Autodesk Fusion 360 part; units mm, degrees
(part 7 of 9)
equation "d395 = ( BaseX + TowerWidth + ModuleGap ) + ( ( ( LeftRun - TowerWidth - ModuleGap ) / 2 ) - DrainWidth / 2 )"
equation "d397 = -( -( ( FootHeight ) + FloorMin + DrainExtension * tan(DrainSlope) + ( ( Depth ) - ( ( Depth ) - Wall ) ) * tan(DrainSlope) ) )"
equation "d398 = ( ( BaseY ) + ( ( Depth ) - Wall ) )"
equation "d399 = -( -( ( FootHeight ) + FloorMin + DrainExtension * tan(DrainSlope) + ( ( Depth ) - ( ( Depth ) + DrainExtension ) ) * tan(DrainSlope) ) )"
equation "d400 = ( ( BaseY ) + ( ( Depth ) + DrainExtension ) )"
equation "d401 = -( -( ( FootHeight ) + PanHeight + 1 mm ) )"
equation "d402 = DrainWidth"
equation "d404 = FootHeight"
equation "d406 = ( BaseX + TowerWidth + ModuleGap ) + ( Wall )"
equation "d407 = ( BaseY ) + ( Wall )"
equation "d410 = PanHeight - DeckThick"
equation "d412 = FootHeight"
equation "d414 = ( BaseX + TowerWidth + ModuleGap ) + ( Wall )"
equation "d415 = ( BaseY ) + ( ( Depth ) - Wall - 12 mm )"
equation "d418 = PanHeight - DeckThick"
equation "d420 = FootHeight"
equation "d422 = ( BaseX + TowerWidth + ModuleGap ) + ( ( LeftRun - TowerWidth - ModuleGap ) - Wall - 12 mm )"
equation "d423 = ( BaseY ) + ( Wall )"
equation "d426 = PanHeight - DeckThick"
equation "d428 = FootHeight"
equation "d430 = ( BaseX + TowerWidth + ModuleGap ) + ( ( LeftRun - TowerWidth - ModuleGap ) - Wall - 12 mm )"
equation "d431 = ( BaseY ) + ( ( Depth ) - Wall - 12 mm )"
equation "d434 = PanHeight - DeckThick"
equation "d436 = ( BaseX + TowerWidth + ModuleGap ) + ( ( ( LeftRun - TowerWidth - ModuleGap ) / 2 ) - DrainWidth / 2 - Wall )"
equation "d438 = -( -( ( FootHeight ) - ( 0.2 mm ) ) )"
equation "d439 = ( ( BaseY ) + ( ( Depth ) + DrainExtension - 2 mm ) )"
equation "d440 = ( ( BaseY ) + ( ( ( Depth ) + DrainExtension - 2 mm ) + ( 1 mm ) ) )"
equation "d441 = -( -( ( FootHeight ) + ( 0.6 mm ) ) )"
equation "d442 = DrainWidth + 2 * Wall"
equation "d444 = FootHeight"
equation "d446 = ( BaseX + TowerWidth + ModuleGap ) + ( ( 11 mm ) - PegSize / 2 - FitClearance )"
equation "d447 = ( BaseY ) + ( ( 11 mm ) - PegSize / 2 - FitClearance )"
equation "d448 = PegSize + 2 * FitClearance"
equation "d449 = PegSize + 2 * FitClearance"
equation "d450 = PegHeight + 0.3 mm"
equation "d452 = FootHeight"
equation "d454 = ( BaseX + TowerWidth + ModuleGap ) + ( ( 11 mm ) - PegSize / 2 - FitClearance )"
equation "d455 = ( BaseY ) + ( ( ( Depth ) - FrontFootInset ) - PegSize / 2 - FitClearance )"
equation "d456 = PegSize + 2 * FitClearance"
equation "d457 = PegSize + 2 * FitClearance"
equation "d458 = PegHeight + 0.3 mm"
equation "d460 = FootHeight"
equation "d462 = ( BaseX + TowerWidth + ModuleGap ) + ( ( ( LeftRun - TowerWidth - ModuleGap ) - 11 mm ) - PegSize / 2 - FitClearance )"
equation "d463 = ( BaseY ) + ( ( 11 mm ) - PegSize / 2 - FitClearance )"
equation "d464 = PegSize + 2 * FitClearance"
equation "d465 = PegSize + 2 * FitClearance"
equation "d466 = PegHeight + 0.3 mm"
equation "d468 = FootHeight"
equation "d470 = ( BaseX + TowerWidth + ModuleGap ) + ( ( ( LeftRun - TowerWidth - ModuleGap ) - 11 mm ) - PegSize / 2 - FitClearance )"
equation "d471 = ( BaseY ) + ( ( ( Depth ) - FrontFootInset ) - PegSize / 2 - FitClearance )"
equation "d472 = PegSize + 2 * FitClearance"
equation "d473 = PegSize + 2 * FitClearance"
equation "d474 = PegHeight + 0.3 mm"
equation "d476 = ( FootHeight ) + PanHeight - DeckThick"
equation "d478 = ( BaseX + TowerWidth + ModuleGap ) + ( Wall + DeckClearance )"
equation "d479 = ( BaseY ) + ( Wall + DeckClearance )"
equation "d480 = ( LeftRun - TowerWidth - ModuleGap ) - 2 * ( Wall + DeckClearance )"
equation "d481 = ( Depth ) - 2 * ( Wall + DeckClearance )"
equation "d482 = DeckThick"
equation "d484 = ( FootHeight ) + PanHeight - DeckThick"
equation "d486 = ( BaseX + TowerWidth + ModuleGap ) + ( ( ( ( LeftRun - TowerWidth - ModuleGap ) - ( 16 * SlotPitch + SlotWidth ) ) / 2 ) + ( 0 * SlotPitch ) )"
equation "d487 = ( BaseY ) + ( Wall + DeckClearance + RimBorder )"
equation "d488 = SlotWidth"
equation "d489 = ( Depth ) - 2 * ( Wall + DeckClearance + RimBorder )"
equation "d490 = DeckThick"
equation "d492 = ( FootHeight ) + PanHeight - DeckThick"
equation "d494 = ( BaseX + TowerWidth + ModuleGap ) + ( ( ( ( LeftRun - TowerWidth - ModuleGap ) - ( 16 * SlotPitch + SlotWidth ) ) / 2 ) + ( 1 * SlotPitch ) )"
equation "d495 = ( BaseY ) + ( Wall + DeckClearance + RimBorder )"
equation "d496 = SlotWidth"
equation "d497 = ( Depth ) - 2 * ( Wall + DeckClearance + RimBorder )"
equation "d498 = DeckThick"
equation "d500 = ( FootHeight ) + PanHeight - DeckThick"
equation "d502 = ( BaseX + TowerWidth + ModuleGap ) + ( ( ( ( LeftRun - TowerWidth - ModuleGap ) - ( 16 * SlotPitch + SlotWidth ) ) / 2 ) + ( 2 * SlotPitch ) )"
equation "d503 = ( BaseY ) + ( Wall + DeckClearance + RimBorder )"
equation "d504 = SlotWidth"
equation "d505 = ( Depth ) - 2 * ( Wall + DeckClearance + RimBorder )"
equation "d506 = DeckThick"
equation "d508 = ( FootHeight ) + PanHeight - DeckThick"
equation "d510 = ( BaseX + TowerWidth + ModuleGap ) + ( ( ( ( LeftRun - TowerWidth - ModuleGap ) - ( 16 * SlotPitch + SlotWidth ) ) / 2 ) + ( 3 * SlotPitch ) )"
equation "d511 = ( BaseY ) + ( Wall + DeckClearance + RimBorder )"
equation "d512 = SlotWidth"
equation "d513 = ( Depth ) - 2 * ( Wall + DeckClearance + RimBorder )"
equation "d514 = DeckThick"
equation "d516 = ( FootHeight ) + PanHeight - DeckThick"
equation "d518 = ( BaseX + TowerWidth + ModuleGap ) + ( ( ( ( LeftRun - TowerWidth - ModuleGap ) - ( 16 * SlotPitch + SlotWidth ) ) / 2 ) + ( 4 * SlotPitch ) )"
equation "d519 = ( BaseY ) + ( Wall + DeckClearance + RimBorder )"
equation "d520 = SlotWidth"
equation "d521 = ( Depth ) - 2 * ( Wall + DeckClearance + RimBorder )"
equation "d522 = DeckThick"
equation "d524 = ( FootHeight ) + PanHeight - DeckThick"
equation "d526 = ( BaseX + TowerWidth + ModuleGap ) + ( ( ( ( LeftRun - TowerWidth - ModuleGap ) - ( 16 * SlotPitch + SlotWidth ) ) / 2 ) + ( 5 * SlotPitch ) )"
equation "d527 = ( BaseY ) + ( Wall + DeckClearance + RimBorder )"
equation "d528 = SlotWidth"
equation "d529 = ( Depth ) - 2 * ( Wall + DeckClearance + RimBorder )"
equation "d530 = DeckThick"
equation "d532 = ( FootHeight ) + PanHeight - DeckThick"
equation "d534 = ( BaseX + TowerWidth + ModuleGap ) + ( ( ( ( LeftRun - TowerWidth - ModuleGap ) - ( 16 * SlotPitch + SlotWidth ) ) / 2 ) + ( 6 * SlotPitch ) )"
equation "d535 = ( BaseY ) + ( Wall + DeckClearance + RimBorder )"
equation "d536 = SlotWidth"
equation "d537 = ( Depth ) - 2 * ( Wall + DeckClearance + RimBorder )"
equation "d538 = DeckThick"
equation "d540 = ( FootHeight ) + PanHeight - DeckThick"
equation "d542 = ( BaseX + TowerWidth + ModuleGap ) + ( ( ( ( LeftRun - TowerWidth - ModuleGap ) - ( 16 * SlotPitch + SlotWidth ) ) / 2 ) + ( 7 * SlotPitch ) )"
equation "d543 = ( BaseY ) + ( Wall + DeckClearance + RimBorder )"
equation "d544 = SlotWidth"
equation "d545 = ( Depth ) - 2 * ( Wall + DeckClearance + RimBorder )"
equation "d546 = DeckThick"
equation "d548 = ( FootHeight ) + PanHeight - DeckThick"
equation "d550 = ( BaseX + TowerWidth + ModuleGap ) + ( ( ( ( LeftRun - TowerWidth - ModuleGap ) - ( 16 * SlotPitch + SlotWidth ) ) / 2 ) + ( 8 * SlotPitch ) )"
equation "d551 = ( BaseY ) + ( Wall + DeckClearance + RimBorder )"
equation "d552 = SlotWidth"
equation "d553 = ( Depth ) - 2 * ( Wall + DeckClearance + RimBorder )"
equation "d554 = DeckThick"
equation "d556 = ( FootHeight ) + PanHeight - DeckThick"
equation "d558 = ( BaseX + TowerWidth + ModuleGap ) + ( ( ( ( LeftRun - TowerWidth - ModuleGap ) - ( 16 * SlotPitch + SlotWidth ) ) / 2 ) + ( 9 * SlotPitch ) )"
equation "d559 = ( BaseY ) + ( Wall + DeckClearance + RimBorder )"
equation "d560 = SlotWidth"
equation "d561 = ( Depth ) - 2 * ( Wall + DeckClearance + RimBorder )"
equation "d562 = DeckThick"
equation "d564 = ( FootHeight ) + PanHeight - DeckThick"
equation "d566 = ( BaseX + TowerWidth + ModuleGap ) + ( ( ( ( LeftRun - TowerWidth - ModuleGap ) - ( 16 * SlotPitch + SlotWidth ) ) / 2 ) + ( 10 * SlotPitch ) )"
equation "d567 = ( BaseY ) + ( Wall + DeckClearance + RimBorder )"
equation "d568 = SlotWidth"
equation "d569 = ( Depth ) - 2 * ( Wall + DeckClearance + RimBorder )"
equation "d570 = DeckThick"
equation "d572 = ( FootHeight ) + PanHeight - DeckThick"
equation "d574 = ( BaseX + TowerWidth + ModuleGap ) + ( ( ( ( LeftRun - TowerWidth - ModuleGap ) - ( 16 * SlotPitch + SlotWidth ) ) / 2 ) + ( 11 * SlotPitch ) )"
equation "d575 = ( BaseY ) + ( Wall + DeckClearance + RimBorder )"
equation "d576 = SlotWidth"
equation "d577 = ( Depth ) - 2 * ( Wall + DeckClearance + RimBorder )"
equation "d578 = DeckThick"
equation "d580 = ( FootHeight ) + PanHeight - DeckThick"
equation "d582 = ( BaseX + TowerWidth + ModuleGap ) + ( ( ( ( LeftRun - TowerWidth - ModuleGap ) - ( 16 * SlotPitch + SlotWidth ) ) / 2 ) + ( 12 * SlotPitch ) )"
equation "d583 = ( BaseY ) + ( Wall + DeckClearance + RimBorder )"
equation "d584 = SlotWidth"
equation "d585 = ( Depth ) - 2 * ( Wall + DeckClearance + RimBorder )"
equation "d586 = DeckThick"
equation "d588 = ( FootHeight ) + PanHeight - DeckThick"
equation "d590 = ( BaseX + TowerWidth + ModuleGap ) + ( ( ( ( LeftRun - TowerWidth - ModuleGap ) - ( 16 * SlotPitch + SlotWidth ) ) / 2 ) + ( 13 * SlotPitch ) )"
equation "d591 = ( BaseY ) + ( Wall + DeckClearance + RimBorder )"
equation "d592 = SlotWidth"
equation "d593 = ( Depth ) - 2 * ( Wall + DeckClearance + RimBorder )"
equation "d594 = DeckThick"
equation "d596 = ( FootHeight ) + PanHeight - DeckThick"
equation "d598 = ( BaseX + TowerWidth + ModuleGap ) + ( ( ( ( LeftRun - TowerWidth - ModuleGap ) - ( 16 * SlotPitch + SlotWidth ) ) / 2 ) + ( 14 * SlotPitch ) )"
equation "d599 = ( BaseY ) + ( Wall + DeckClearance + RimBorder )"
equation "d600 = SlotWidth"
equation "d601 = ( Depth ) - 2 * ( Wall + DeckClearance + RimBorder )"
equation "d602 = DeckThick"
equation "d604 = ( FootHeight ) + PanHeight - DeckThick"
equation "d606 = ( BaseX + TowerWidth + ModuleGap ) + ( ( ( ( LeftRun - TowerWidth - ModuleGap ) - ( 16 * SlotPitch + SlotWidth ) ) / 2 ) + ( 15 * SlotPitch ) )"
equation "d607 = ( BaseY ) + ( Wall + DeckClearance + RimBorder )"
equation "d608 = SlotWidth"
equation "d609 = ( Depth ) - 2 * ( Wall + DeckClearance + RimBorder )"
equation "d610 = DeckThick"
equation "d612 = ( FootHeight ) + PanHeight - DeckThick"
equation "d614 = ( BaseX + TowerWidth + ModuleGap ) + ( ( ( ( LeftRun - TowerWidth - ModuleGap ) - ( 16 * SlotPitch + SlotWidth ) ) / 2 ) + ( 16 * SlotPitch ) )"
equation "d615 = ( BaseY ) + ( Wall + DeckClearance + RimBorder )"
equation "d616 = SlotWidth"
equation "d617 = ( Depth ) - 2 * ( Wall + DeckClearance + RimBorder )"
equation "d618 = DeckThick"
equation "d620 = ( FootHeight ) + PanHeight - DeckThick"
equation "d622 = ( BaseX + TowerWidth + ModuleGap ) + ( ( LeftRun - TowerWidth - ModuleGap ) / 2 - 8 mm )"
equation "d623 = ( BaseY ) + ( ( Depth ) - Wall - DeckClearance - 4 mm )"
equation "d626 = DeckThick"
equation "d630 = ( BaseX + TowerWidth + ModuleGap ) + ( ( 11 mm ) - FootSize / 2 )"
equation "d631 = ( BaseY ) + ( ( 11 mm ) - FootSize / 2 )"
equation "d632 = FootSize"
equation "d633 = FootSize"
equation "d634 = FootHeight"
equation "d636 = FootHeight"
equation "d638 = ( BaseX + TowerWidth + ModuleGap ) + ( ( 11 mm ) - PegSize / 2 )"
equation "d639 = ( BaseY ) + ( ( 11 mm ) - PegSize / 2 )"
equation "d640 = PegSize"
equation "d641 = PegSize"
equation "d642 = PegHeight"
equation "d646 = ( BaseX + TowerWidth + ModuleGap ) + ( ( 11 mm ) - FootSize / 2 )"
equation "d647 = ( BaseY ) + ( ( ( Depth ) - FrontFootInset ) - FootSize / 2 )"
equation "d648 = FootSize"
equation "d649 = FootSize"
equation "d650 = FootHeight"
equation "d652 = FootHeight"
equation "d654 = ( BaseX + TowerWidth + ModuleGap ) + ( ( 11 mm ) - PegSize / 2 )"
equation "d655 = ( BaseY ) + ( ( ( Depth ) - FrontFootInset ) - PegSize / 2 )"
equation "d656 = PegSize"
equation "d657 = PegSize"
equation "d658 = PegHeight"
equation "d662 = ( BaseX + TowerWidth + ModuleGap ) + ( ( ( LeftRun - TowerWidth - ModuleGap ) - 11 mm ) - FootSize / 2 )"
equation "d663 = ( BaseY ) + ( ( 11 mm ) - FootSize / 2 )"
equation "d664 = FootSize"
equation "d665 = FootSize"
equation "d666 = FootHeight"
equation "d668 = FootHeight"
equation "d670 = ( BaseX + TowerWidth + ModuleGap ) + ( ( ( LeftRun - TowerWidth - ModuleGap ) - 11 mm ) - PegSize / 2 )"
equation "d671 = ( BaseY ) + ( ( 11 mm ) - PegSize / 2 )"
equation "d672 = PegSize"
equation "d673 = PegSize"
equation "d674 = PegHeight"
equation "d678 = ( BaseX + TowerWidth + ModuleGap ) + ( ( ( LeftRun - TowerWidth - ModuleGap ) - 11 mm ) - FootSize / 2 )"
equation "d679 = ( BaseY ) + ( ( ( Depth ) - FrontFootInset ) - FootSize / 2 )"
equation "d680 = FootSize"
equation "d681 = FootSize"
equation "d682 = FootHeight"
equation "d684 = FootHeight"
equation "d686 = ( BaseX + TowerWidth + ModuleGap ) + ( ( ( LeftRun - TowerWidth - ModuleGap ) - 11 mm ) - PegSize / 2 )"
equation "d687 = ( BaseY ) + ( ( ( Depth ) - FrontFootInset ) - PegSize / 2 )"
equation "d688 = PegSize"
equation "d689 = PegSize"
equation "d690 = PegHeight"
equation "d692 = FootHeight"
equation "d694 = ( BaseX + LeftRun + FaucetGap ) + ( 0 mm )"
equation "d695 = ( BaseY ) + ( 0 mm )"
equation "d696 = ( RightRun - ModuleGap ) / 2"
equation "d697 = Depth"
equation "d698 = PanHeight"
equation "d702 = ( BaseX + LeftRun + FaucetGap ) + ( Wall )"
equation "d704 = -( -( ( FootHeight ) + FloorMin + DrainExtension * tan(DrainSlope) + ( ( Depth ) - ( Wall ) ) * tan(DrainSlope) ) )"
equation "d705 = ( ( BaseY ) + ( Wall ) )"
equation "d706 = -( -( ( FootHeight ) + FloorMin + DrainExtension * tan(DrainSlope) + ( ( Depth ) - ( ( Depth ) - Wall ) ) * tan(DrainSlope) ) )"
equation "d707 = ( ( BaseY ) + ( ( Depth ) - Wall ) )"
equation "d708 = -( -( ( FootHeight ) + PanHeight + 1 mm ) )"
equation "d709 = ( ( RightRun - ModuleGap ) / 2 ) - 2 * Wall"
equation "d711 = ( BaseX + LeftRun + FaucetGap ) + ( ( ( RightRun - ModuleGap ) / 4 ) - DrainWidth / 2 - Wall )"
equation "d713 = -( -( FootHeight ) )"
equation "d714 = ( ( BaseY ) + ( ( Depth ) - Wall ) )"
equation "d715 = ( ( BaseY ) + ( ( Depth ) + DrainExtension ) )"
equation "d716 = -( -( ( FootHeight ) + FloorMin + DrainExtension * tan(DrainSlope) + ( ( Depth ) - ( ( Depth ) + DrainExtension ) ) * tan(DrainSlope) ) )"
equation "d717 = -( -( ( FootHeight ) + FloorMin + DrainExtension * tan(DrainSlope) + ( ( Depth ) - ( ( Depth ) - Wall ) ) * tan(DrainSlope) ) )"
equation "d718 = DrainWidth + 2 * Wall"
equation "d720 = ( BaseX + LeftRun + FaucetGap ) + ( ( ( RightRun - ModuleGap ) / 4 ) - DrainWidth / 2 - Wall )"
equation "d722 = -( -( FootHeight ) )"
equation "d723 = ( ( BaseY ) + ( ( Depth ) - Wall ) )"
equation "d724 = ( ( BaseY ) + ( ( Depth ) + DrainExtension ) )"
equation "d725 = -( -( ( ( FootHeight ) + FloorMin + DrainExtension * tan(DrainSlope) + ( ( Depth ) - ( ( Depth ) + DrainExtension ) ) * tan(DrainSlope) ) + ( 6 mm ) ) )"
equation "d726 = -( -( ( ( FootHeight ) + FloorMin + DrainExtension * tan(DrainSlope) + ( ( Depth ) - ( ( Depth ) - Wall ) ) * tan(DrainSlope) ) + ( 6 mm ) ) )"
equation "d727 = Wall"
equation "d729 = ( BaseX + LeftRun + FaucetGap ) + ( ( ( RightRun - ModuleGap ) / 4 ) + DrainWidth / 2 )"
equation "d731 = -( -( FootHeight ) )"
equation "d732 = ( ( BaseY ) + ( ( Depth ) - Wall ) )"
equation "d733 = ( ( BaseY ) + ( ( Depth ) + DrainExtension ) )"
equation "d734 = -( -( ( ( FootHeight ) + FloorMin + DrainExtension * tan(DrainSlope) + ( ( Depth ) - ( ( Depth ) + DrainExtension ) ) * tan(DrainSlope) ) + ( 6 mm ) ) )"
equation "d735 = -( -( ( ( FootHeight ) + FloorMin + DrainExtension * tan(DrainSlope) + ( ( Depth ) - ( ( Depth ) - Wall ) ) * tan(DrainSlope) ) + ( 6 mm ) ) )"
equation "d736 = Wall"
equation "d738 = ( BaseX + LeftRun + FaucetGap ) + ( ( ( RightRun - ModuleGap ) / 4 ) - DrainWidth / 2 )"
equation "d740 = -( -( ( FootHeight ) + FloorMin + DrainExtension * tan(DrainSlope) + ( ( Depth ) - ( ( Depth ) - Wall ) ) * tan(DrainSlope) ) )"
equation "d741 = ( ( BaseY ) + ( ( Depth ) - Wall ) )"
equation "d742 = -( -( ( FootHeight ) + FloorMin + DrainExtension * tan(DrainSlope) + ( ( Depth ) - ( ( Depth ) + DrainExtension ) ) * tan(DrainSlope) ) )"
equation "d743 = ( ( BaseY ) + ( ( Depth ) + DrainExtension ) )"
equation "d744 = -( -( ( FootHeight ) + PanHeight + 1 mm ) )"
equation "d745 = DrainWidth"
equation "d747 = FootHeight"
equation "d749 = ( BaseX + LeftRun + FaucetGap ) + ( Wall )"
equation "d750 = ( BaseY ) + ( Wall )"
equation "d753 = PanHeight - DeckThick"
equation "d755 = FootHeight"
equation "d757 = ( BaseX + LeftRun + FaucetGap ) + ( Wall )"
equation "d758 = ( BaseY ) + ( ( Depth ) - Wall - 12 mm )"
equation "d761 = PanHeight - DeckThick"
equation "d763 = FootHeight"
equation "d765 = ( BaseX + LeftRun + FaucetGap ) + ( ( ( RightRun - ModuleGap ) / 2 ) - Wall - 12 mm )"
equation "d766 = ( BaseY ) + ( Wall )"
equation "d769 = PanHeight - DeckThick"
equation "d771 = FootHeight"
equation "d773 = ( BaseX + LeftRun + FaucetGap ) + ( ( ( RightRun - ModuleGap ) / 2 ) - Wall - 12 mm )"
equation "d774 = ( BaseY ) + ( ( Depth ) - Wall - 12 mm )"
equation "d777 = PanHeight - DeckThick"
equation "d779 = ( BaseX + LeftRun + FaucetGap ) + ( ( ( RightRun - ModuleGap ) / 4 ) - DrainWidth / 2 - Wall )"
equation "d781 = -( -( ( FootHeight ) - ( 0.2 mm ) ) )"
equation "d782 = ( ( BaseY ) + ( ( Depth ) + DrainExtension - 2 mm ) )"
equation "d783 = ( ( BaseY ) + ( ( ( Depth ) + DrainExtension - 2 mm ) + ( 1 mm ) ) )"
equation "d784 = -( -( ( FootHeight ) + ( 0.6 mm ) ) )"
equation "d785 = DrainWidth + 2 * Wall"
equation "d787 = FootHeight"
equation "d789 = ( BaseX + LeftRun + FaucetGap ) + ( ( 11 mm ) - PegSize / 2 - FitClearance )"
equation "d790 = ( BaseY ) + ( ( 11 mm ) - PegSize / 2 - FitClearance )"
equation "d791 = PegSize + 2 * FitClearance"
equation "d792 = PegSize + 2 * FitClearance"
equation "d793 = PegHeight + 0.3 mm"
equation "d795 = FootHeight"
equation "d797 = ( BaseX + LeftRun + FaucetGap ) + ( ( 11 mm ) - PegSize / 2 - FitClearance )"
equation "d798 = ( BaseY ) + ( ( ( Depth ) - FrontFootInset ) - PegSize / 2 - FitClearance )"
equation "d799 = PegSize + 2 * FitClearance"
equation "d800 = PegSize + 2 * FitClearance"
equation "d801 = PegHeight + 0.3 mm"
equation "d803 = FootHeight"
equation "d805 = ( BaseX + LeftRun + FaucetGap ) + ( ( ( ( RightRun - ModuleGap ) / 2 ) - 11 mm ) - PegSize / 2 - FitClearance )"
equation "d806 = ( BaseY ) + ( ( 11 mm ) - PegSize / 2 - FitClearance )"
equation "d807 = PegSize + 2 * FitClearance"
equation "d808 = PegSize + 2 * FitClearance"
equation "d809 = PegHeight + 0.3 mm"
equation "d811 = FootHeight"
equation "d813 = ( BaseX + LeftRun + FaucetGap ) + ( ( ( ( RightRun - ModuleGap ) / 2 ) - 11 mm ) - PegSize / 2 - FitClearance )"
equation "d814 = ( BaseY ) + ( ( ( Depth ) - FrontFootInset ) - PegSize / 2 - FitClearance )"
equation "d815 = PegSize + 2 * FitClearance"
equation "d816 = PegSize + 2 * FitClearance"
equation "d817 = PegHeight + 0.3 mm"
equation "d819 = ( FootHeight ) + PanHeight - DeckThick"
equation "d821 = ( BaseX + LeftRun + FaucetGap ) + ( Wall + DeckClearance )"
equation "d822 = ( BaseY ) + ( Wall + DeckClearance )"
equation "d823 = ( ( RightRun - ModuleGap ) / 2 ) - 2 * ( Wall + DeckClearance )"
equation "d824 = ( Depth ) - 2 * ( Wall + DeckClearance )"
equation "d825 = DeckThick"
equation "d827 = ( FootHeight ) + PanHeight - DeckThick"
equation "d829 = ( BaseX + LeftRun + FaucetGap ) + ( ( ( ( ( RightRun - ModuleGap ) / 2 ) - ( 10 * SlotPitch + SlotWidth ) ) / 2 ) + ( 0 * SlotPitch ) )"
equation "d830 = ( BaseY ) + ( Wall + DeckClearance + RimBorder )"
equation "d831 = SlotWidth"
equation "d832 = ( Depth ) - 2 * ( Wall + DeckClearance + RimBorder )"
equation "d833 = DeckThick"
equation "d835 = ( FootHeight ) + PanHeight - DeckThick"
equation "d837 = ( BaseX + LeftRun + FaucetGap ) + ( ( ( ( ( RightRun - ModuleGap ) / 2 ) - ( 10 * SlotPitch + SlotWidth ) ) / 2 ) + ( 1 * SlotPitch ) )"
equation "d838 = ( BaseY ) + ( Wall + DeckClearance + RimBorder )"
equation "d839 = SlotWidth"
equation "d840 = ( Depth ) - 2 * ( Wall + DeckClearance + RimBorder )"
equation "d841 = DeckThick"
equation "d843 = ( FootHeight ) + PanHeight - DeckThick"
equation "d845 = ( BaseX + LeftRun + FaucetGap ) + ( ( ( ( ( RightRun - ModuleGap ) / 2 ) - ( 10 * SlotPitch + SlotWidth ) ) / 2 ) + ( 2 * SlotPitch ) )"
equation "d846 = ( BaseY ) + ( Wall + DeckClearance + RimBorder )"
equation "d847 = SlotWidth"
equation "d848 = ( Depth ) - 2 * ( Wall + DeckClearance + RimBorder )"
equation "d849 = DeckThick"
equation "d851 = ( FootHeight ) + PanHeight - DeckThick"
equation "d853 = ( BaseX + LeftRun + FaucetGap ) + ( ( ( ( ( RightRun - ModuleGap ) / 2 ) - ( 10 * SlotPitch + SlotWidth ) ) / 2 ) + ( 3 * SlotPitch ) )"
equation "d854 = ( BaseY ) + ( Wall + DeckClearance + RimBorder )"
equation "d855 = SlotWidth"
equation "d856 = ( Depth ) - 2 * ( Wall + DeckClearance + RimBorder )"
equation "d857 = DeckThick"
equation "d859 = ( FootHeight ) + PanHeight - DeckThick"
equation "d861 = ( BaseX + LeftRun + FaucetGap ) + ( ( ( ( ( RightRun - ModuleGap ) / 2 ) - ( 10 * SlotPitch + SlotWidth ) ) / 2 ) + ( 4 * SlotPitch ) )"
equation "d862 = ( BaseY ) + ( Wall + DeckClearance + RimBorder )"
equation "d863 = SlotWidth"
equation "d864 = ( Depth ) - 2 * ( Wall + DeckClearance + RimBorder )"
equation "d865 = DeckThick"
equation "d867 = ( FootHeight ) + PanHeight - DeckThick"
equation "d869 = ( BaseX + LeftRun + FaucetGap ) + ( ( ( ( ( RightRun - ModuleGap ) / 2 ) - ( 10 * SlotPitch + SlotWidth ) ) / 2 ) + ( 5 * SlotPitch ) )"
equation "d870 = ( BaseY ) + ( Wall + DeckClearance + RimBorder )"
equation "d871 = SlotWidth"
equation "d872 = ( Depth ) - 2 * ( Wall + DeckClearance + RimBorder )"
equation "d873 = DeckThick"
equation "d875 = ( FootHeight ) + PanHeight - DeckThick"
equation "d877 = ( BaseX + LeftRun + FaucetGap ) + ( ( ( ( ( RightRun - ModuleGap ) / 2 ) - ( 10 * SlotPitch + SlotWidth ) ) / 2 ) + ( 6 * SlotPitch ) )"
equation "d878 = ( BaseY ) + ( Wall + DeckClearance + RimBorder )"
equation "d879 = SlotWidth"
equation "d880 = ( Depth ) - 2 * ( Wall + DeckClearance + RimBorder )"
equation "d881 = DeckThick"
equation "d883 = ( FootHeight ) + PanHeight - DeckThick"
equation "d885 = ( BaseX + LeftRun + FaucetGap ) + ( ( ( ( ( RightRun - ModuleGap ) / 2 ) - ( 10 * SlotPitch + SlotWidth ) ) / 2 ) + ( 7 * SlotPitch ) )"
equation "d886 = ( BaseY ) + ( Wall + DeckClearance + RimBorder )"
equation "d887 = SlotWidth"
equation "d888 = ( Depth ) - 2 * ( Wall + DeckClearance + RimBorder )"
equation "d889 = DeckThick"
equation "d891 = ( FootHeight ) + PanHeight - DeckThick"
equation "d893 = ( BaseX + LeftRun + FaucetGap ) + ( ( ( ( ( RightRun - ModuleGap ) / 2 ) - ( 10 * SlotPitch + SlotWidth ) ) / 2 ) + ( 8 * SlotPitch ) )"
equation "d894 = ( BaseY ) + ( Wall + DeckClearance + RimBorder )"
equation "d895 = SlotWidth"
equation "d896 = ( Depth ) - 2 * ( Wall + DeckClearance + RimBorder )"
equation "d897 = DeckThick"
equation "d899 = ( FootHeight ) + PanHeight - DeckThick"
equation "d901 = ( BaseX + LeftRun + FaucetGap ) + ( ( ( ( ( RightRun - ModuleGap ) / 2 ) - ( 10 * SlotPitch + SlotWidth ) ) / 2 ) + ( 9 * SlotPitch ) )"
equation "d902 = ( BaseY ) + ( Wall + DeckClearance + RimBorder )"
equation "d903 = SlotWidth"
equation "d904 = ( Depth ) - 2 * ( Wall + DeckClearance + RimBorder )"
equation "d905 = DeckThick"
equation "d907 = ( FootHeight ) + PanHeight - DeckThick"
equation "d909 = ( BaseX + LeftRun + FaucetGap ) + ( ( ( ( ( RightRun - ModuleGap ) / 2 ) - ( 10 * SlotPitch + SlotWidth ) ) / 2 ) + ( 10 * SlotPitch ) )"
equation "d910 = ( BaseY ) + ( Wall + DeckClearance + RimBorder )"
equation "d911 = SlotWidth"
equation "d912 = ( Depth ) - 2 * ( Wall + DeckClearance + RimBorder )"
equation "d913 = DeckThick"
equation "d915 = ( FootHeight ) + PanHeight - DeckThick"
equation "d917 = ( BaseX + LeftRun + FaucetGap ) + ( ( ( RightRun - ModuleGap ) / 2 ) / 2 - 8 mm )"
equation "d918 = ( BaseY ) + ( ( Depth ) - Wall - DeckClearance - 4 mm )"
equation "d921 = DeckThick"
equation "d925 = ( BaseX + LeftRun + FaucetGap ) + ( ( 11 mm ) - FootSize / 2 )"
equation "d926 = ( BaseY ) + ( ( 11 mm ) - FootSize / 2 )"
equation "d927 = FootSize"
equation "d928 = FootSize"
equation "d929 = FootHeight"
equation "d931 = FootHeight"
equation "d933 = ( BaseX + LeftRun + FaucetGap ) + ( ( 11 mm ) - PegSize / 2 )"
equation "d934 = ( BaseY ) + ( ( 11 mm ) - PegSize / 2 )"
equation "d935 = PegSize"
equation "d936 = PegSize"
equation "d937 = PegHeight"
equation "d941 = ( BaseX + LeftRun + FaucetGap ) + ( ( 11 mm ) - FootSize / 2 )"
equation "d942 = ( BaseY ) + ( ( ( Depth ) - FrontFootInset ) - FootSize / 2 )"
equation "d943 = FootSize"
equation "d944 = FootSize"
equation "d945 = FootHeight"
equation "d947 = FootHeight"
equation "d949 = ( BaseX + LeftRun + FaucetGap ) + ( ( 11 mm ) - PegSize / 2 )"
equation "d950 = ( BaseY ) + ( ( ( Depth ) - FrontFootInset ) - PegSize / 2 )"
equation "d951 = PegSize"
equation "d952 = PegSize"
equation "d953 = PegHeight"
equation "d957 = ( BaseX + LeftRun + FaucetGap ) + ( ( ( ( RightRun - ModuleGap ) / 2 ) - 11 mm ) - FootSize / 2 )"
equation "d958 = ( BaseY ) + ( ( 11 mm ) - FootSize / 2 )"
equation "d959 = FootSize"
equation "d960 = FootSize"
equation "d961 = FootHeight"
equation "d963 = FootHeight"
equation "d965 = ( BaseX + LeftRun + FaucetGap ) + ( ( ( ( RightRun - ModuleGap ) / 2 ) - 11 mm ) - PegSize / 2 )"
equation "d966 = ( BaseY ) + ( ( 11 mm ) - PegSize / 2 )"
equation "d967 = PegSize"
equation "d968 = PegSize"
equation "d969 = PegHeight"
equation "d973 = ( BaseX + LeftRun + FaucetGap ) + ( ( ( ( RightRun - ModuleGap ) / 2 ) - 11 mm ) - FootSize / 2 )"
equation "d974 = ( BaseY ) + ( ( ( Depth ) - FrontFootInset ) - FootSize / 2 )"
equation "d975 = FootSize"
equation "d976 = FootSize"
equation "d977 = FootHeight"
equation "d979 = FootHeight"
equation "d981 = ( BaseX + LeftRun + FaucetGap ) + ( ( ( ( RightRun - ModuleGap ) / 2 ) - 11 mm ) - PegSize / 2 )"
equation "d982 = ( BaseY ) + ( ( ( Depth ) - FrontFootInset ) - PegSize / 2 )"
equation "d983 = PegSize"
equation "d984 = PegSize"
equation "d985 = PegHeight"
equation "d987 = FootHeight"
equation "d989 = ( BaseX + LeftRun + FaucetGap + ( RightRun + ModuleGap ) / 2 ) + ( 0 mm )"
equation "d990 = ( BaseY ) + ( 0 mm )"
equation "d991 = ( RightRun - ModuleGap ) / 2"
equation "d992 = Depth"
equation "d993 = PanHeight"
equation "d997 = ( BaseX + LeftRun + FaucetGap + ( RightRun + ModuleGap ) / 2 ) + ( Wall )"
equation "d999 = -( -( ( FootHeight ) + FloorMin + DrainExtension * tan(DrainSlope) + ( ( Depth ) - ( Wall ) ) * tan(DrainSlope) ) )"
equation "d1000 = ( ( BaseY ) + ( Wall ) )"
equation "d1001 = -( -( ( FootHeight ) + FloorMin + DrainExtension * tan(DrainSlope) + ( ( Depth ) - ( ( Depth ) - Wall ) ) * tan(DrainSlope) ) )"
equation "d1002 = ( ( BaseY ) + ( ( Depth ) - Wall ) )"
equation "d1003 = -( -( ( FootHeight ) + PanHeight + 1 mm ) )"
equation "d1004 = ( ( RightRun - ModuleGap ) / 2 ) - 2 * Wall"
equation "d1006 = ( BaseX + LeftRun + FaucetGap + ( RightRun + ModuleGap ) / 2 ) + ( ( 18 mm ) - DrainWidth / 2 - Wall )"
equation "d1008 = -( -( FootHeight ) )"
equation "d1009 = ( ( BaseY ) + ( ( Depth ) - Wall ) )"
equation "d1010 = ( ( BaseY ) + ( ( Depth ) + DrainExtension ) )"
equation "d1011 = -( -( ( FootHeight ) + FloorMin + DrainExtension * tan(DrainSlope) + ( ( Depth ) - ( ( Depth ) + DrainExtension ) ) * tan(DrainSlope) ) )"
equation "d1012 = -( -( ( FootHeight ) + FloorMin + DrainExtension * tan(DrainSlope) + ( ( Depth ) - ( ( Depth ) - Wall ) ) * tan(DrainSlope) ) )"
equation "d1013 = DrainWidth + 2 * Wall"
equation "d1015 = ( BaseX + LeftRun + FaucetGap + ( RightRun + ModuleGap ) / 2 ) + ( ( 18 mm ) - DrainWidth / 2 - Wall )"
equation "d1017 = -( -( FootHeight ) )"
equation "d1018 = ( ( BaseY ) + ( ( Depth ) - Wall ) )"
equation "d1019 = ( ( BaseY ) + ( ( Depth ) + DrainExtension ) )"
equation "d1020 = -( -( ( ( FootHeight ) + FloorMin + DrainExtension * tan(DrainSlope) + ( ( Depth ) - ( ( Depth ) + DrainExtension ) ) * tan(DrainSlope) ) + ( 6 mm ) ) )"
equation "d1021 = -( -( ( ( FootHeight ) + FloorMin + DrainExtension * tan(DrainSlope) + ( ( Depth ) - ( ( Depth ) - Wall ) ) * tan(DrainSlope) ) + ( 6 mm ) ) )"
equation "d1022 = Wall"
equation "d1024 = ( BaseX + LeftRun + FaucetGap + ( RightRun + ModuleGap ) / 2 ) + ( ( 18 mm ) + DrainWidth / 2 )"
equation "d1026 = -( -( FootHeight ) )"
equation "d1027 = ( ( BaseY ) + ( ( Depth ) - Wall ) )"
equation "d1028 = ( ( BaseY ) + ( ( Depth ) + DrainExtension ) )"
equation "d1029 = -( -( ( ( FootHeight ) + FloorMin + DrainExtension * tan(DrainSlope) + ( ( Depth ) - ( ( Depth ) + DrainExtension ) ) * tan(DrainSlope) ) + ( 6 mm ) ) )"
equation "d1030 = -( -( ( ( FootHeight ) + FloorMin + DrainExtension * tan(DrainSlope) + ( ( Depth ) - ( ( Depth ) - Wall ) ) * tan(DrainSlope) ) + ( 6 mm ) ) )"
equation "d1031 = Wall"
equation "d1033 = ( BaseX + LeftRun + FaucetGap + ( RightRun + ModuleGap ) / 2 ) + ( ( 18 mm ) - DrainWidth / 2 )"
equation "d1035 = -( -( ( FootHeight ) + FloorMin + DrainExtension * tan(DrainSlope) + ( ( Depth ) - ( ( Depth ) - Wall ) ) * tan(DrainSlope) ) )"
equation "d1036 = ( ( BaseY ) + ( ( Depth ) - Wall ) )"
equation "d1037 = -( -( ( FootHeight ) + FloorMin + DrainExtension * tan(DrainSlope) + ( ( Depth ) - ( ( Depth ) + DrainExtension ) ) * tan(DrainSlope) ) )"
equation "d1038 = ( ( BaseY ) + ( ( Depth ) + DrainExtension ) )"
equation "d1039 = -( -( ( FootHeight ) + PanHeight + 1 mm ) )"
equation "d1040 = DrainWidth"
equation "d1042 = FootHeight"
equation "d1044 = ( BaseX + LeftRun + FaucetGap + ( RightRun + ModuleGap ) / 2 ) + ( Wall )"
equation "d1045 = ( BaseY ) + ( Wall )"
equation "d1048 = PanHeight - DeckThick"
equation "d1050 = FootHeight"
equation "d1052 = ( BaseX + LeftRun + FaucetGap + ( RightRun + ModuleGap ) / 2 ) + ( ( 18 mm ) + DrainWidth / 2 + 3 mm )"
equation "d1053 = ( BaseY ) + ( ( Depth ) - Wall - 12 mm )"
equation "d1056 = PanHeight - DeckThick"
equation "d1058 = FootHeight"
equation "d1060 = ( BaseX + LeftRun + FaucetGap + ( RightRun + ModuleGap ) / 2 ) + ( ( ( RightRun - ModuleGap ) / 2 ) - Wall - 12 mm )"
equation "d1061 = ( BaseY ) + ( Wall )"
equation "d1064 = PanHeight - DeckThick"
equation "d1066 = FootHeight"
equation "d1068 = ( BaseX + LeftRun + FaucetGap + ( RightRun + ModuleGap ) / 2 ) + ( ( ( RightRun - ModuleGap ) / 2 ) - Wall - 12 mm )"
equation "d1069 = ( BaseY ) + ( ( Depth ) - Wall - 12 mm )"
equation "d1072 = PanHeight - DeckThick"
equation "d1074 = ( BaseX + LeftRun + FaucetGap + ( RightRun + ModuleGap ) / 2 ) + ( ( 18 mm ) - DrainWidth / 2 - Wall )"
equation "d1076 = -( -( ( FootHeight ) - ( 0.2 mm ) ) )"
equation "d1077 = ( ( BaseY ) + ( ( Depth ) + DrainExtension - 2 mm ) )"
equation "d1078 = ( ( BaseY ) + ( ( ( Depth ) + DrainExtension - 2 mm ) + ( 1 mm ) ) )"
equation "d1079 = -( -( ( FootHeight ) + ( 0.6 mm ) ) )"
equation "d1080 = DrainWidth + 2 * Wall"
equation "d1082 = FootHeight"
equation "d1084 = ( BaseX + LeftRun + FaucetGap + ( RightRun + ModuleGap ) / 2 ) + ( ( 11 mm ) - PegSize / 2 - FitClearance )"
equation "d1085 = ( BaseY ) + ( ( 11 mm ) - PegSize / 2 - FitClearance )"
equation "d1086 = PegSize + 2 * FitClearance"
equation "d1087 = PegSize + 2 * FitClearance"
equation "d1088 = PegHeight + 0.3 mm"
equation "d1090 = FootHeight"
equation "d1092 = ( BaseX + LeftRun + FaucetGap + ( RightRun + ModuleGap ) / 2 ) + ( ( 11 mm ) - PegSize / 2 - FitClearance )"
equation "d1093 = ( BaseY ) + ( ( ( Depth ) - FrontFootInset ) - PegSize / 2 - FitClearance )"
equation "d1094 = PegSize + 2 * FitClearance"
equation "d1095 = PegSize + 2 * FitClearance"
equation "d1096 = PegHeight + 0.3 mm"
equation "d1098 = FootHeight"
equation "d1100 = ( BaseX + LeftRun + FaucetGap + ( RightRun + ModuleGap ) / 2 ) + ( ( ( ( RightRun - ModuleGap ) / 2 ) - 11 mm ) - PegSize / 2 - FitClearance )"
equation "d1101 = ( BaseY ) + ( ( 11 mm ) - PegSize / 2 - FitClearance )"
equation "d1102 = PegSize + 2 * FitClearance"
equation "d1103 = PegSize + 2 * FitClearance"
equation "d1104 = PegHeight + 0.3 mm"
equation "d1106 = FootHeight"
equation "d1108 = ( BaseX + LeftRun + FaucetGap + ( RightRun + ModuleGap ) / 2 ) + ( ( ( ( RightRun - ModuleGap ) / 2 ) - 11 mm ) - PegSize / 2 - FitClearance )"
equation "d1109 = ( BaseY ) + ( ( ( Depth ) - FrontFootInset ) - PegSize / 2 - FitClearance )"
equation "d1110 = PegSize + 2 * FitClearance"
equation "d1111 = PegSize + 2 * FitClearance"
equation "d1112 = PegHeight + 0.3 mm"
equation "d1114 = ( FootHeight ) + PanHeight - DeckThick"
equation "d1116 = ( BaseX + LeftRun + FaucetGap + ( RightRun + ModuleGap ) / 2 ) + ( Wall + DeckClearance )"
equation "d1117 = ( BaseY ) + ( Wall + DeckClearance )"
equation "d1118 = ( ( RightRun - ModuleGap ) / 2 ) - 2 * ( Wall + DeckClearance )"
equation "d1119 = ( Depth ) - 2 * ( Wall + DeckClearance )"
equation "d1120 = DeckThick"
equation "d1122 = ( FootHeight ) + PanHeight - DeckThick"
equation "d1124 = ( BaseX + LeftRun + FaucetGap + ( RightRun + ModuleGap ) / 2 ) + ( ( ( ( ( RightRun - ModuleGap ) / 2 ) - ( 10 * SlotPitch + SlotWidth ) ) / 2 ) + ( 0 * SlotPitch ) )"
equation "d1125 = ( BaseY ) + ( Wall + DeckClearance + RimBorder )"
equation "d1126 = SlotWidth"
equation "d1127 = ( Depth ) - 2 * ( Wall + DeckClearance + RimBorder )"
equation "d1128 = DeckThick"
equation "d1130 = ( FootHeight ) + PanHeight - DeckThick"
equation "d1132 = ( BaseX + LeftRun + FaucetGap + ( RightRun + ModuleGap ) / 2 ) + ( ( ( ( ( RightRun - ModuleGap ) / 2 ) - ( 10 * SlotPitch + SlotWidth ) ) / 2 ) + ( 1 * SlotPitch ) )"
equation "d1133 = ( BaseY ) + ( Wall + DeckClearance + RimBorder )"
equation "d1134 = SlotWidth"
equation "d1135 = ( Depth ) - 2 * ( Wall + DeckClearance + RimBorder )"
equation "d1136 = DeckThick"
equation "d1138 = ( FootHeight ) + PanHeight - DeckThick"
equation "d1140 = ( BaseX + LeftRun + FaucetGap + ( RightRun + ModuleGap ) / 2 ) + ( ( ( ( ( RightRun - ModuleGap ) / 2 ) - ( 10 * SlotPitch + SlotWidth ) ) / 2 ) + ( 2 * SlotPitch ) )"
equation "d1141 = ( BaseY ) + ( Wall + DeckClearance + RimBorder )"
equation "d1142 = SlotWidth"
equation "d1143 = ( Depth ) - 2 * ( Wall + DeckClearance + RimBorder )"
equation "d1144 = DeckThick"
equation "d1146 = ( FootHeight ) + PanHeight - DeckThick"
equation "d1148 = ( BaseX + LeftRun + FaucetGap + ( RightRun + ModuleGap ) / 2 ) + ( ( ( ( ( RightRun - ModuleGap ) / 2 ) - ( 10 * SlotPitch + SlotWidth ) ) / 2 ) + ( 3 * SlotPitch ) )"
equation "d1149 = ( BaseY ) + ( Wall + DeckClearance + RimBorder )"
equation "d1150 = SlotWidth"
equation "d1151 = ( Depth ) - 2 * ( Wall + DeckClearance + RimBorder )"
equation "d1152 = DeckThick"
equation "d1154 = ( FootHeight ) + PanHeight - DeckThick"
equation "d1156 = ( BaseX + LeftRun + FaucetGap + ( RightRun + ModuleGap ) / 2 ) + ( ( ( ( ( RightRun - ModuleGap ) / 2 ) - ( 10 * SlotPitch + SlotWidth ) ) / 2 ) + ( 4 * SlotPitch ) )"
equation "d1157 = ( BaseY ) + ( Wall + DeckClearance + RimBorder )"
equation "d1158 = SlotWidth"
equation "d1159 = ( Depth ) - 2 * ( Wall + DeckClearance + RimBorder )"
equation "d1160 = DeckThick"
equation "d1162 = ( FootHeight ) + PanHeight - DeckThick"
equation "d1164 = ( BaseX + LeftRun + FaucetGap + ( RightRun + ModuleGap ) / 2 ) + ( ( ( ( ( RightRun - ModuleGap ) / 2 ) - ( 10 * SlotPitch + SlotWidth ) ) / 2 ) + ( 5 * SlotPitch ) )"
equation "d1165 = ( BaseY ) + ( Wall + DeckClearance + RimBorder )"
equation "d1166 = SlotWidth"
equation "d1167 = ( Depth ) - 2 * ( Wall + DeckClearance + RimBorder )"
equation "d1168 = DeckThick"
equation "d1170 = ( FootHeight ) + PanHeight - DeckThick"
equation "d1172 = ( BaseX + LeftRun + FaucetGap + ( RightRun + ModuleGap ) / 2 ) + ( ( ( ( ( RightRun - ModuleGap ) / 2 ) - ( 10 * SlotPitch + SlotWidth ) ) / 2 ) + ( 6 * SlotPitch ) )"
equation "d1173 = ( BaseY ) + ( Wall + DeckClearance + RimBorder )"
equation "d1174 = SlotWidth"
equation "d1175 = ( Depth ) - 2 * ( Wall + DeckClearance + RimBorder )"
equation "d1176 = DeckThick"
equation "d1178 = ( FootHeight ) + PanHeight - DeckThick"
equation "d1180 = ( BaseX + LeftRun + FaucetGap + ( RightRun + ModuleGap ) / 2 ) + ( ( ( ( ( RightRun - ModuleGap ) / 2 ) - ( 10 * SlotPitch + SlotWidth ) ) / 2 ) + ( 7 * SlotPitch ) )"
equation "d1181 = ( BaseY ) + ( Wall + DeckClearance + RimBorder )"
equation "d1182 = SlotWidth"
equation "d1183 = ( Depth ) - 2 * ( Wall + DeckClearance + RimBorder )"
equation "d1184 = DeckThick"
equation "d1186 = ( FootHeight ) + PanHeight - DeckThick"
equation "d1188 = ( BaseX + LeftRun + FaucetGap + ( RightRun + ModuleGap ) / 2 ) + ( ( ( ( ( RightRun - ModuleGap ) / 2 ) - ( 10 * SlotPitch + SlotWidth ) ) / 2 ) + ( 8 * SlotPitch ) )"
equation "d1189 = ( BaseY ) + ( Wall + DeckClearance + RimBorder )"
equation "d1190 = SlotWidth"
equation "d1191 = ( Depth ) - 2 * ( Wall + DeckClearance + RimBorder )"
equation "d1192 = DeckThick"
equation "d1194 = ( FootHeight ) + PanHeight - DeckThick"
equation "d1196 = ( BaseX + LeftRun + FaucetGap + ( RightRun + ModuleGap ) / 2 ) + ( ( ( ( ( RightRun - ModuleGap ) / 2 ) - ( 10 * SlotPitch + SlotWidth ) ) / 2 ) + ( 9 * SlotPitch ) )"
equation "d1197 = ( BaseY ) + ( Wall + DeckClearance + RimBorder )"
equation "d1198 = SlotWidth"
equation "d1199 = ( Depth ) - 2 * ( Wall + DeckClearance + RimBorder )"
equation "d1200 = DeckThick"
equation "d1202 = ( FootHeight ) + PanHeight - DeckThick"
equation "d1204 = ( BaseX + LeftRun + FaucetGap + ( RightRun + ModuleGap ) / 2 ) + ( ( ( ( ( RightRun - ModuleGap ) / 2 ) - ( 10 * SlotPitch + SlotWidth ) ) / 2 ) + ( 10 * SlotPitch ) )"
equation "d1205 = ( BaseY ) + ( Wall + DeckClearance + RimBorder )"
equation "d1206 = SlotWidth"
equation "d1207 = ( Depth ) - 2 * ( Wall + DeckClearance + RimBorder )"
equation "d1208 = DeckThick"
equation "d1210 = ( FootHeight ) + PanHeight - DeckThick"
equation "d1212 = ( BaseX + LeftRun + FaucetGap + ( RightRun + ModuleGap ) / 2 ) + ( ( ( RightRun - ModuleGap ) / 2 ) / 2 - 8 mm )"
equation "d1213 = ( BaseY ) + ( ( Depth ) - Wall - DeckClearance - 4 mm )"
equation "d1216 = DeckThick"
equation "d1220 = ( BaseX + LeftRun + FaucetGap + ( RightRun + ModuleGap ) / 2 ) + ( ( 11 mm ) - FootSize / 2 )"
equation "d1221 = ( BaseY ) + ( ( 11 mm ) - FootSize / 2 )"
equation "d1222 = FootSize"
equation "d1223 = FootSize"
equation "d1224 = FootHeight"
equation "d1226 = FootHeight"
equation "d1228 = ( BaseX + LeftRun + FaucetGap + ( RightRun + ModuleGap ) / 2 ) + ( ( 11 mm ) - PegSize / 2 )"
equation "d1229 = ( BaseY ) + ( ( 11 mm ) - PegSize / 2 )"
equation "d1230 = PegSize"
equation "d1231 = PegSize"
equation "d1232 = PegHeight"
equation "d1236 = ( BaseX + LeftRun + FaucetGap + ( RightRun + ModuleGap ) / 2 ) + ( ( 11 mm ) - FootSize / 2 )"
equation "d1237 = ( BaseY ) + ( ( ( Depth ) - FrontFootInset ) - FootSize / 2 )"
equation "d1238 = FootSize"
equation "d1239 = FootSize"
equation "d1240 = FootHeight"
equation "d1242 = FootHeight"
equation "d1244 = ( BaseX + LeftRun + FaucetGap + ( RightRun + ModuleGap ) / 2 ) + ( ( 11 mm ) - PegSize / 2 )"
equation "d1245 = ( BaseY ) + ( ( ( Depth ) - FrontFootInset ) - PegSize / 2 )"
equation "d1246 = PegSize"
equation "d1247 = PegSize"
equation "d1248 = PegHeight"
equation "d1252 = ( BaseX + LeftRun + FaucetGap + ( RightRun + ModuleGap ) / 2 ) + ( ( ( ( RightRun - ModuleGap ) / 2 ) - 11 mm ) - FootSize / 2 )"
equation "d1253 = ( BaseY ) + ( ( 11 mm ) - FootSize / 2 )"
equation "d1254 = FootSize"
equation "d1255 = FootSize"
equation "d1256 = FootHeight"
equation "d1258 = FootHeight"
equation "d1260 = ( BaseX + LeftRun + FaucetGap + ( RightRun + ModuleGap ) / 2 ) + ( ( ( ( RightRun - ModuleGap ) / 2 ) - 11 mm ) - PegSize / 2 )"
equation "d1261 = ( BaseY ) + ( ( 11 mm ) - PegSize / 2 )"
equation "d1262 = PegSize"
equation "d1263 = PegSize"
equation "d1264 = PegHeight"
equation "d1268 = ( BaseX + LeftRun + FaucetGap + ( RightRun + ModuleGap ) / 2 ) + ( ( ( ( RightRun - ModuleGap ) / 2 ) - 11 mm ) - FootSize / 2 )"
equation "d1269 = ( BaseY ) + ( ( ( Depth ) - FrontFootInset ) - FootSize / 2 )"
equation "d1270 = FootSize"
equation "d1271 = FootSize"
equation "d1272 = FootHeight"
equation "d1274 = FootHeight"
equation "d1276 = ( BaseX + LeftRun + FaucetGap + ( RightRun + ModuleGap ) / 2 ) + ( ( ( ( RightRun - ModuleGap ) / 2 ) - 11 mm ) - PegSize / 2 )"
equation "d1277 = ( BaseY ) + ( ( ( Depth ) - FrontFootInset ) - PegSize / 2 )"
equation "d1278 = PegSize"
equation "d1279 = PegSize"
equation "d1280 = PegHeight"
equation "d1282 = FootHeight"
equation "d1284 = ( BaseX ) + ( 0 mm )"
equation "d1285 = ( BaseY + Depth + ModuleGap ) + ( ( LeftReach ) - ( ( 0 mm ) + ( LeftReach ) ) )"
equation "d1286 = LeftSideDepth"
equation "d1287 = LeftReach"
equation "d1288 = PanHeight"
equation "d1292 = ( BaseY + Depth + ModuleGap ) + ( ( LeftReach ) - ( Wall ) )"
equation "d1294 = ( ( BaseX ) + ( Wall ) )"
equation "d1295 = -( -( ( FootHeight ) + FloorMin + DrainExtension * tan(DrainSlope) + ( ( LeftSideDepth ) - ( Wall ) ) * tan(DrainSlope) ) )"
equation "d1296 = ( ( BaseX ) + ( ( LeftSideDepth ) - Wall ) )"
equation "d1297 = -( -( ( FootHeight ) + FloorMin + DrainExtension * tan(DrainSlope) + ( ( LeftSideDepth ) - ( ( LeftSideDepth ) - Wall ) ) * tan(DrainSlope) ) )"
equation "d1298 = -( -( ( FootHeight ) + PanHeight + 1 mm ) )"
equation "d1299 = -( -( -( ( LeftReach ) - 2 * Wall ) ) )"
equation "d1301 = ( BaseY + Depth + ModuleGap ) + ( ( LeftReach ) - ( ( LeftReach / 2 ) - DrainWidth / 2 - Wall ) )"
equation "d1303 = ( ( BaseX ) + ( ( LeftSideDepth ) - Wall ) )"
equation "d1304 = -( -( FootHeight ) )"
equation "d1305 = ( ( BaseX ) + ( ( LeftSideDepth ) + DrainExtension ) )"
equation "d1306 = -( -( ( FootHeight ) + FloorMin + DrainExtension * tan(DrainSlope) + ( ( LeftSideDepth ) - ( ( LeftSideDepth ) + DrainExtension ) ) * tan(DrainSlope) ) )"
equation "d1307 = -( -( ( FootHeight ) + FloorMin + DrainExtension * tan(DrainSlope) + ( ( LeftSideDepth ) - ( ( LeftSideDepth ) - Wall ) ) * tan(DrainSlope) ) )"
equation "d1308 = -( DrainWidth + 2 * Wall )"
equation "d1310 = ( BaseY + Depth + ModuleGap ) + ( ( LeftReach ) - ( ( LeftReach / 2 ) - DrainWidth / 2 - Wall ) )"
equation "d1312 = ( ( BaseX ) + ( ( LeftSideDepth ) - Wall ) )"
equation "d1313 = -( -( FootHeight ) )"
equation "d1314 = ( ( BaseX ) + ( ( LeftSideDepth ) + DrainExtension ) )"
equation "d1315 = -( -( ( ( FootHeight ) + FloorMin + DrainExtension * tan(DrainSlope) + ( ( LeftSideDepth ) - ( ( LeftSideDepth ) + DrainExtension ) ) * tan(DrainSlope) ) + ( 6 mm ) ) )"
equation "d1316 = -( -( ( ( FootHeight ) + FloorMin + DrainExtension * tan(DrainSlope) + ( ( LeftSideDepth ) - ( ( LeftSideDepth ) - Wall ) ) * tan(DrainSlope) ) + ( 6 mm ) ) )"
equation "d1317 = -( Wall )"
equation "d1319 = ( BaseY + Depth + ModuleGap ) + ( ( LeftReach ) - ( ( LeftReach / 2 ) + DrainWidth / 2 ) )"
equation "d1321 = ( ( BaseX ) + ( ( LeftSideDepth ) - Wall ) )"
equation "d1322 = -( -( FootHeight ) )"
equation "d1323 = ( ( BaseX ) + ( ( LeftSideDepth ) + DrainExtension ) )"
equation "d1324 = -( -( ( ( FootHeight ) + FloorMin + DrainExtension * tan(DrainSlope) + ( ( LeftSideDepth ) - ( ( LeftSideDepth ) + DrainExtension ) ) * tan(DrainSlope) ) + ( 6 mm ) ) )"
equation "d1325 = -( -( ( ( FootHeight ) + FloorMin + DrainExtension * tan(DrainSlope) + ( ( LeftSideDepth ) - ( ( LeftSideDepth ) - Wall ) ) * tan(DrainSlope) ) + ( 6 mm ) ) )"
equation "d1326 = -( Wall )"
equation "d1328 = ( BaseY + Depth + ModuleGap ) + ( ( LeftReach ) - ( ( LeftReach / 2 ) - DrainWidth / 2 ) )"
equation "d1330 = ( ( BaseX ) + ( ( LeftSideDepth ) - Wall ) )"
equation "d1331 = -( -( ( FootHeight ) + FloorMin + DrainExtension * tan(DrainSlope) + ( ( LeftSideDepth ) - ( ( LeftSideDepth ) - Wall ) ) * tan(DrainSlope) ) )"
equation "d1332 = ( ( BaseX ) + ( ( LeftSideDepth ) + DrainExtension ) )"
equation "d1333 = -( -( ( FootHeight ) + FloorMin + DrainExtension * tan(DrainSlope) + ( ( LeftSideDepth ) - ( ( LeftSideDepth ) + DrainExtension ) ) * tan(DrainSlope) ) )"
equation "d1334 = -( -( ( FootHeight ) + PanHeight + 1 mm ) )"
equation "d1335 = -( -( -( DrainWidth ) ) )"
equation "d1337 = FootHeight"
equation "d1339 = ( BaseX ) + ( Wall )"
equation "d1340 = ( BaseY + Depth + ModuleGap ) + ( ( LeftReach ) - ( ( Wall ) + ( 12 mm ) ) )"
equation "d1343 = PanHeight - DeckThick"
equation "d1345 = FootHeight"
equation "d1347 = ( BaseX ) + ( ( LeftSideDepth ) - Wall - 12 mm )"
equation "d1348 = ( BaseY + Depth + ModuleGap ) + ( ( LeftReach ) - ( ( Wall ) + ( 12 mm ) ) )"
equation "d1351 = PanHeight - DeckThick"
equation "d1353 = FootHeight"
equation "d1355 = ( BaseX ) + ( Wall )"
equation "d1356 = ( BaseY + Depth + ModuleGap ) + ( ( LeftReach ) - ( ( ( LeftReach ) - Wall - 12 mm ) + ( 12 mm ) ) )"
equation "d1359 = PanHeight - DeckThick"
equation "d1361 = FootHeight"
equation "d1363 = ( BaseX ) + ( ( LeftSideDepth ) - Wall - 12 mm )"
equation "d1364 = ( BaseY + Depth + ModuleGap ) + ( ( LeftReach ) - ( ( ( LeftReach ) - Wall - 12 mm ) + ( 12 mm ) ) )"
equation "d1367 = PanHeight - DeckThick"
equation "d1369 = ( BaseY + Depth + ModuleGap ) + ( ( LeftReach ) - ( ( LeftReach / 2 ) - DrainWidth / 2 - Wall ) )"
equation "d1371 = ( ( BaseX ) + ( ( LeftSideDepth ) + DrainExtension - 2 mm ) )"
equation "d1372 = -( -( ( FootHeight ) - ( 0.2 mm ) ) )"
equation "d1373 = ( ( BaseX ) + ( ( ( LeftSideDepth ) + DrainExtension - 2 mm ) + ( 1 mm ) ) )"
equation "d1374 = -( -( ( FootHeight ) + ( 0.6 mm ) ) )"
equation "d1375 = -( -( -( DrainWidth + 2 * Wall ) ) )"
equation "d1377 = FootHeight"
equation "d1379 = ( BaseX ) + ( ( 11 mm ) - PegSize / 2 - FitClearance )"
equation "d1380 = ( BaseY + Depth + ModuleGap ) + ( ( LeftReach ) - ( ( ( 11 mm ) - PegSize / 2 - FitClearance ) + ( PegSize + 2 * FitClearance ) ) )"
equation "d1381 = PegSize + 2 * FitClearance"
equation "d1382 = PegSize + 2 * FitClearance"
equation "d1383 = PegHeight + 0.3 mm"
equation "d1385 = FootHeight"
equation "d1387 = ( BaseX ) + ( ( ( LeftSideDepth ) - FrontFootInset ) - PegSize / 2 - FitClearance )"
equation "d1388 = ( BaseY + Depth + ModuleGap ) + ( ( LeftReach ) - ( ( ( 11 mm ) - PegSize / 2 - FitClearance ) + ( PegSize + 2 * FitClearance ) ) )"
equation "d1389 = PegSize + 2 * FitClearance"
equation "d1390 = PegSize + 2 * FitClearance"
equation "d1391 = PegHeight + 0.3 mm"
equation "d1393 = FootHeight"
equation "d1395 = ( BaseX ) + ( ( 11 mm ) - PegSize / 2 - FitClearance )"
equation "d1396 = ( BaseY + Depth + ModuleGap ) + ( ( LeftReach ) - ( ( ( ( LeftReach ) - 11 mm ) - PegSize / 2 - FitClearance ) + ( PegSize + 2 * FitClearance ) ) )"
equation "d1397 = PegSize + 2 * FitClearance"
equation "d1398 = PegSize + 2 * FitClearance"
equation "d1399 = PegHeight + 0.3 mm"
equation "d1401 = FootHeight"
equation "d1403 = ( BaseX ) + ( ( ( LeftSideDepth ) - FrontFootInset ) - PegSize / 2 - FitClearance )"
equation "d1404 = ( BaseY + Depth + ModuleGap ) + ( ( LeftReach ) - ( ( ( ( LeftReach ) - 11 mm ) - PegSize / 2 - FitClearance ) + ( PegSize + 2 * FitClearance ) ) )"
equation "d1405 = PegSize + 2 * FitClearance"
equation "d1406 = PegSize + 2 * FitClearance"
equation "d1407 = PegHeight + 0.3 mm"
equation "d1409 = ( FootHeight ) + PanHeight - DeckThick"
equation "d1411 = ( BaseX ) + ( Wall + DeckClearance )"
equation "d1412 = ( BaseY + Depth + ModuleGap ) + ( ( LeftReach ) - ( ( Wall + DeckClearance ) + ( ( LeftReach ) - 2 * ( Wall + DeckClearance ) ) ) )"
equation "d1413 = ( LeftSideDepth ) - 2 * ( Wall + DeckClearance )"
equation "d1414 = ( LeftReach ) - 2 * ( Wall + DeckClearance )"
equation "d1415 = DeckThick"
equation "d1417 = ( FootHeight ) + PanHeight - DeckThick"
equation "d1419 = ( BaseX ) + ( Wall + DeckClearance + RimBorder )"
equation "d1420 = ( BaseY + Depth + ModuleGap ) + ( ( LeftReach ) - ( ( ( ( ( LeftReach ) - ( 14 * SlotPitch + SlotWidth ) ) / 2 ) + ( 0 * SlotPitch ) ) + ( SlotWidth ) ) )"
equation "d1421 = ( LeftSideDepth ) - 2 * ( Wall + DeckClearance + RimBorder )"
equation "d1422 = SlotWidth"
equation "d1423 = DeckThick"
equation "d1425 = ( FootHeight ) + PanHeight - DeckThick"
equation "d1427 = ( BaseX ) + ( Wall + DeckClearance + RimBorder )"
equation "d1428 = ( BaseY + Depth + ModuleGap ) + ( ( LeftReach ) - ( ( ( ( ( LeftReach ) - ( 14 * SlotPitch + SlotWidth ) ) / 2 ) + ( 1 * SlotPitch ) ) + ( SlotWidth ) ) )"
equation "d1429 = ( LeftSideDepth ) - 2 * ( Wall + DeckClearance + RimBorder )"
equation "d1430 = SlotWidth"
equation "d1431 = DeckThick"
equation "d1433 = ( FootHeight ) + PanHeight - DeckThick"
equation "d1435 = ( BaseX ) + ( Wall + DeckClearance + RimBorder )"
equation "d1436 = ( BaseY + Depth + ModuleGap ) + ( ( LeftReach ) - ( ( ( ( ( LeftReach ) - ( 14 * SlotPitch + SlotWidth ) ) / 2 ) + ( 2 * SlotPitch ) ) + ( SlotWidth ) ) )"
equation "d1437 = ( LeftSideDepth ) - 2 * ( Wall + DeckClearance + RimBorder )"
equation "d1438 = SlotWidth"
equation "d1439 = DeckThick"
equation "d1441 = ( FootHeight ) + PanHeight - DeckThick"
equation "d1443 = ( BaseX ) + ( Wall + DeckClearance + RimBorder )"
equation "d1444 = ( BaseY + Depth + ModuleGap ) + ( ( LeftReach ) - ( ( ( ( ( LeftReach ) - ( 14 * SlotPitch + SlotWidth ) ) / 2 ) + ( 3 * SlotPitch ) ) + ( SlotWidth ) ) )"
equation "d1445 = ( LeftSideDepth ) - 2 * ( Wall + DeckClearance + RimBorder )"
equation "d1446 = SlotWidth"
equation "d1447 = DeckThick"
equation "d1449 = ( FootHeight ) + PanHeight - DeckThick"
equation "d1451 = ( BaseX ) + ( Wall + DeckClearance + RimBorder )"
equation "d1452 = ( BaseY + Depth + ModuleGap ) + ( ( LeftReach ) - ( ( ( ( ( LeftReach ) - ( 14 * SlotPitch + SlotWidth ) ) / 2 ) + ( 4 * SlotPitch ) ) + ( SlotWidth ) ) )"
equation "d1453 = ( LeftSideDepth ) - 2 * ( Wall + DeckClearance + RimBorder )"
equation "d1454 = SlotWidth"
equation "d1455 = DeckThick"
equation "d1457 = ( FootHeight ) + PanHeight - DeckThick"